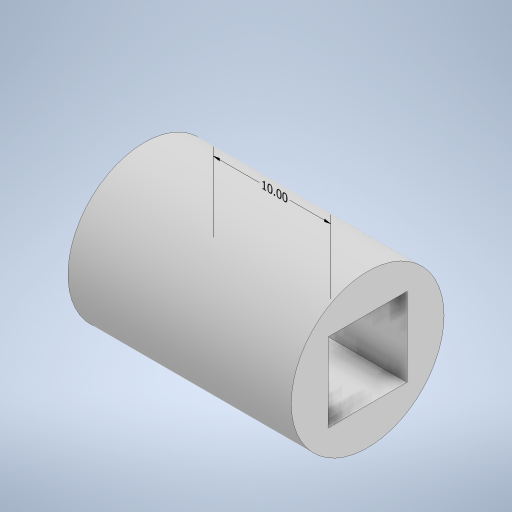
# Autodesk Inventor part: Adaptador
Saved by Autodesk Inventor 2023 (Build 270158000, 158)
## iProperties
Created: 2023-06-06
Part Number: Adaptador
Material: Genérico
Document SubType Name: Modeling
Designer: sergi
Density: 1 g/cm^3
Appearance: Valor por defecto
Author: sergi
Autodesk Inventor part; units mm, degrees
ref_plane "YZ Plane" through (0, 0, 0) normal (1, 0, 0) x (0, 1, 0)
ref_plane "XZ Plane" through (0, 0, 0) normal (0, 1, 0) x (-1, 0, 0)
ref_plane "XY Plane" through (0, 0, 0) normal (0, 0, 1) x (1, 0, 0)
sketch "Boceto1" plane through (0, 0, 0) normal (1, 0, 0) x (0, 1, 0)
  circle A0 centre (0, 0) radius 2.9
  line L0 (2.2, 1.8894) -> (2.2, -1.8894)
  line L1 (-2.2, 1.8894) -> (-2.2, -1.8894)
  circle A1 centre (0, 0) radius 6.5
  dimension "d0" = 5.8
  dimension "d1" = 2.2
  dimension "d2" = 2.2
  dimension "d3" = 13
  constraints: 4 end point, 4 point on circle, 2 centre point, 2 coincident, 1 parallel, 1 vertical
  measures "d0" diameter of A0
  measures "d1" distance from line of L0 point (0, 0)
  measures "d2" distance from line of point (0, 0) L1
  measures "d3" diameter of A1
extrude "Extrusión1" add sketch "Boceto1" along normal blind 9 contours A0 L0 | L1 A0 | A1
sketch "Boceto2" plane through (9, 0, 0) normal (1, 0, 0) x (0, 0, -1)
  circle A0 centre (0, 0) radius 6.5
  line L0 (3.35, -3.35) -> (-3.35, -3.35)
  line L1 (-3.35, -3.35) -> (-3.35, 3.35)
  line L2 (-3.35, 3.35) -> (3.35, 3.35)
  line L3 (3.35, 3.35) -> (3.35, -3.35)
  line L4 (3.35, -3.35) -> (-3.35, 3.35) construction
  line L5 (-3.35, -3.35) -> (3.35, 3.35) construction
  dimension "d6" = 6.7
  dimension "d7" = 6.7
  constraints: 12 end point, 2 midpoint, 2 parallel, 1 centre point, 1 coincident, 1 horizontal, 1 perpendicular
  measures "d6" distance of L1.end L2.end
  measures "d7" distance of L0.end L1.end
extrude "Extrusión2" add sketch "Boceto2" along normal blind 10
